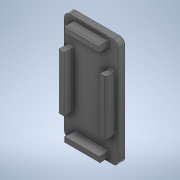
# Autodesk Inventor part: SP18V1 Tapacanto Superior
Saved by Autodesk Inventor 2021.2 (Build 252289000, 289)
## iProperties
Created: 2026-06-08
Part Number: SP18V1 Tapacanto Superior
Material: ABS Plastic
Document SubType Name: Modeling
Designer: NELSON
Density: 1.06 g/cm^3
Appearance: Smooth - Black
Author: NELSON
Autodesk Inventor part; units mm, degrees
ref_plane "YZ Plane" through (0, 0, 0) normal (1, 0, 0) x (0, 1, 0)
ref_plane "XZ Plane" through (0, 0, 0) normal (0, 1, 0) x (-1, 0, 0)
ref_plane "XY Plane" through (0, 0, 0) normal (0, 0, 1) x (1, 0, 0)
sketch "Boceto1" plane through (0, 0, 0) normal (0, 0, 1) x (1, 0, 0)
  line L0 (20, -40) -> (-20, -40)
  line L1 (-20, -40) -> (-20, 40)
  line L2 (-20, 40) -> (20, 40)
  line L3 (20, 40) -> (20, -40)
  line L4 (20, -40) -> (-20, 40) construction
  line L5 (-20, -40) -> (20, 40) construction
  point P0 (0, 0)
  dimension "d0" = 40
  dimension "d22" = 80
  constraints: 12 end point, 2 midpoint, 2 parallel, 1 horizontal, 1 perpendicular
  measures "d0" distance of L1.end L2.end
  measures "d22" distance of L0.end L1.end
extrude "Extrusión1" add sketch "Boceto1" along normal blind 5
sketch "Boceto2" plane through (0, 0, 5) normal (0, 0, 1) x (1, 0, 0)
  line L0 (-17.76, -37.76) -> (17.76, -37.76)
  line L1 (17.76, -37.76) -> (17.76, 37.76)
  line L2 (17.76, 37.76) -> (-17.76, 37.76)
  line L3 (-17.76, 37.76) -> (-17.76, -37.76)
  line L4 (-17.76, -37.76) -> (17.76, 37.76) construction
  line L5 (17.76, -37.76) -> (-17.76, 37.76) construction
  line L6 (-17.36, 37.36) -> (17.36, 37.36)
  line L7 (17.36, 37.36) -> (17.36, -37.36)
  line L8 (17.36, -37.36) -> (-17.36, -37.36)
  line L9 (-17.36, -37.36) -> (-17.36, 37.36)
  line L10 (-17.36, 0) -> (-15.36, 0)
  line L11 (-13.36, -20) -> (-17.36, -20)
  line L12 (-17.36, -20) -> (-17.36, 20)
  line L13 (-17.36, 20) -> (-13.36, 20)
  line L14 (-13.36, 20) -> (-13.36, -20)
  line L15 (-13.36, -20) -> (-17.36, 20) construction
  line L16 (-17.36, -20) -> (-13.36, 20) construction
  line L17 (0, 0) -> (0, 2.694)
  line L18 (0, 0) -> (-1.9567, 0)
  line L19 (13.36, -20) -> (17.36, -20)
  line L20 (17.36, -20) -> (17.36, 20)
  line L21 (17.36, 20) -> (13.36, 20)
  line L22 (13.36, 20) -> (13.36, -20)
  line L23 (13.36, -20) -> (17.36, 20) construction
  line L24 (17.36, -20) -> (13.36, 20) construction
  line L25 (0, 37.36) -> (0, 35.36)
  line L26 (-12.5, 33.36) -> (12.5, 33.36)
  line L27 (12.5, 33.36) -> (12.5, 37.36)
  line L28 (12.5, 37.36) -> (-12.5, 37.36)
  line L29 (-12.5, 37.36) -> (-12.5, 33.36)
  line L30 (-12.5, 33.36) -> (12.5, 37.36) construction
  line L31 (12.5, 33.36) -> (-12.5, 37.36) construction
  line L32 (-12.5, -33.36) -> (12.5, -33.36)
  line L33 (12.5, -33.36) -> (12.5, -37.36)
  line L34 (12.5, -37.36) -> (-12.5, -37.36)
  line L35 (-12.5, -37.36) -> (-12.5, -33.36)
  line L36 (-12.5, -33.36) -> (12.5, -37.36) construction
  line L37 (12.5, -33.36) -> (-12.5, -37.36) construction
  point P0 (15.36, 0)
  point P1 (0, -35.36)
  dimension "d27" = 35.52
  dimension "d28" = 75.52
  dimension "d29" = 0.4
  dimension "d30" = 2
  dimension "d31" = 40
  dimension "d32" = 2
  dimension "d33" = 25
  constraints: 76 end point, 12 midpoint, 10 symmetric about line, 8 parallel, 5 horizontal, 4 perpendicular, 2 point on line, 2 vertical, 3 other
  measures "d27" distance of L2.end L1.end
  measures "d28" distance of L1.end L0.end
  measures "d29" distance between parallel lines of L2 L6
  measures "d30" distance of L10.start L10.end
  measures "d31" distance of L11.end L12.end
  measures "d32" distance of L25.start L25.end
  measures "d33" distance of L28.end L27.end
extrude "Extrusión2" add sketch "Boceto2" along normal blind 7 draft 2 contours L6 L27 L26 L29 | L13 L14 L11 L9 | L7 L19 L22 L21 | L35 L32 L33 L8
fillet "Empalme3" radius 4 4 edges at (20, 40, 2.5) (-20, 40, 2.5) (20, -40, 2.5) (-20, -40, 2.5)
fillet "Empalme3" radius 1 16 edges at (12.5, 35.36, 5) (0, 33.36, 5) (-12.5, 35.36, 5) (-17.6044, 0, 12) (0, 37.6044, 12) (-15.36, 20, 5) (-13.36, 0, 5) (-15.36, -20, 5) (15.36, -20, 5) (15.36, 20, 5) (17.6044, 0, 12) (13.36, 0, 5) (0, -33.36, 5) (12.5, -35.36, 5) (0, -37.6044, 12) (-12.5, -35.36, 5)
chamfer "Chamfer1" distance 0.3 angle 45 8 edges at (0, 40, 0) (-18.8284, 38.8284, 0) (-20, 0, 0) (-18.8284, -38.8284, 0) (0, -40, 0) (18.8284, -38.8284, 0) (20, 0, 0) (18.8284, 38.8284, 0)
